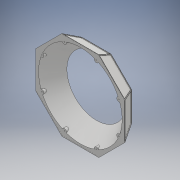
# Autodesk Inventor part: meteostanica radiation shield zakladna
Saved by Autodesk Inventor 2017 (Build 210142000, 142)
## iProperties
Created: 2017-02-23
Part Number: meteostanica radiation shield zakladna
Material: Generic
Document SubType Name: Modeling
Designer: Luc3as
Density: 1 g/cm^3
Appearance: Default
Author: Luc3as
Autodesk Inventor part; units mm, degrees
ref_plane "YZ Plane" through (0, 0, 0) normal (1, 0, 0) x (0, 1, 0)
ref_plane "XZ Plane" through (0, 0, 0) normal (0, 1, 0) x (-1, 0, 0)
ref_plane "XY Plane" through (0, 0, 0) normal (0, 0, 1) x (1, 0, 0)
sketch "Sketch1" plane through (0, 0, 0) normal (0, 1, 0) x (-1, 0, 0)
  circle A0 centre (0, 0) radius 75
  line L0 (82.6875, -34.2503) -> (34.2503, -82.6875)
  line L1 (34.2503, -82.6875) -> (-34.2503, -82.6875)
  line L2 (-34.2503, -82.6875) -> (-82.6875, -34.2503)
  line L3 (-82.6875, -34.2503) -> (-82.6875, 34.2503)
  line L4 (-82.6875, 34.2503) -> (-34.2503, 82.6875)
  line L5 (-34.2503, 82.6875) -> (34.2503, 82.6875)
  line L6 (34.2503, 82.6875) -> (82.6875, 34.2503)
  line L7 (82.6875, 34.2503) -> (82.6875, -34.2503)
  circle A1 centre (0, 0) radius 55
  line L8 (63.0062, -26.098) -> (26.098, -63.0062)
  line L9 (26.098, -63.0062) -> (-26.098, -63.0062)
  line L10 (-26.098, -63.0062) -> (-63.0062, -26.098)
  line L11 (-63.0062, -26.098) -> (-63.0062, 26.098)
  line L12 (-63.0062, 26.098) -> (-26.098, 63.0062)
  line L13 (-26.098, 63.0062) -> (26.098, 63.0062)
  line L14 (26.098, 63.0062) -> (63.0062, 26.098)
  line L15 (63.0062, 26.098) -> (63.0062, -26.098)
  point P0 (75, 0)
  dimension "d0" = 150
  dimension "d1" = 110
  constraints: 32 end point, 3 coincident, 1 centre point, 1 horizontal alignment, 3 other
  measures "d1" diameter of A1
extrude "Extrusion1" add sketch "Sketch1" along normal blind 30 contours A0 | L0 L1 L2 L3 L4 L5 L6 L7 | L8 L9 L10 L11 L12 L13 L14 L15
draft "FaceDraft1" angle 30 pull direction (0, 1, 0) faces at (-50.396, 20, 66.5418) (11.4168, 20, 82.6875) (66.5418, 20, 50.396) (-82.6875, 10, 11.4168) (-66.5418, 10, -50.396) (-11.4168, 10, -82.6875) (50.396, 10, -66.5418) (82.6875, 10, -11.4168) fixed edges at (-58.4689, 0, 58.4689) (0, 0, 82.6875) (58.4689, 0, 58.4689) (-82.6875, 0, 0) (-58.4689, 0, -58.4689) (0, 0, -82.6875) (58.4689, 0, -58.4689) (82.6875, 0, 0)
sketch "Sketch2" plane through (82.6875, 0, -34.2503) normal (0.6123724, 0.5, -0.6123724) x (-0.7071068, 0, -0.7071068)
  line L0 (68.5006, 0) -> (0, 0) projected
  line L1 (34.2503, 0) -> (61.2503, 0)
  line L2 (61.2503, 0) -> (61.2503, 27)
  line L3 (61.2503, 27) -> (7.2503, 27)
  line L4 (7.2503, 27) -> (7.2503, 0)
  line L5 (7.2503, 0) -> (34.2503, 0)
  line L6 (68.5006, 0) -> (61.3262, 34.641) projected
  line L7 (68.5006, 0) -> (0, 0) projected
  line L8 (68.5006, 0) -> (61.3262, 34.641) projected
  line L9 (7.1744, 34.641) -> (61.3262, 34.641) projected
  line L10 (0, 0) -> (7.1744, 34.641) projected
  line L11 (60.5121, 33.641) -> (67.2722, 1)
  line L12 (67.2722, 1) -> (1.2283, 1)
  line L13 (1.2283, 1) -> (7.9885, 33.641)
  line L14 (7.9885, 33.641) -> (60.5121, 33.641)
  point P0 (34.2503, 41.3438)
  dimension "d5" = 27
  dimension "d6" = 27
  dimension "d7" = 54
  dimension "d10" = 1
  constraints: 18 end point, 4 perpendicular, 2 point on line, 1 midpoint, 3 other
  measures "d5" distance of L1.start L1.end
  measures "d6" distance of L1.end L2.end
  measures "d7" distance of L2.end L3.end
  measures "d10" distance between parallel lines of L9 L14
draft "FaceDraft2" angle 37 pull direction (0, -1, 0) faces at (50.386, 20, -22.0512) fixed edges at (55, 30, 0)
sketch "Sketch3" plane through (82.6875, 0, 34.2503) normal (0.8660254, 0.5, 0) x (0, 0, -1)
  line L0 (7.1744, 34.641) -> (61.3262, 34.641) projected
  line L1 (68.5006, 0) -> (0, 0) projected
  line L2 (68.5006, 0) -> (61.3262, 34.641) projected
  line L3 (7.1744, 34.641) -> (61.3262, 34.641) projected
  line L4 (0, 0) -> (7.1744, 34.641) projected
  line L5 (60.5121, 33.641) -> (67.2722, 1)
  line L6 (67.2722, 1) -> (1.2283, 1)
  line L7 (1.2283, 1) -> (7.9885, 33.641)
  line L8 (7.9885, 33.641) -> (60.5121, 33.641)
  point P0 (34.2503, 41.3437)
  dimension "d9" = 1
  constraints: 8 end point, 3 other
  measures "d9" distance between parallel lines of L2 L5
sketch "Sketch4" plane through (82.6875, 0, -34.2503) normal (0.6123724, 0.5, -0.6123724) x (-0.7071068, 0, -0.7071068)
  point P0 (34.2503, 41.3438)
sketch "Sketch5" plane through (34.2503, 0, -82.6875) normal (0, 0.5, -0.8660254) x (-1, 0, 0)
  line L0 (7.1744, 34.641) -> (61.3262, 34.641) projected
  line L1 (68.5006, 0) -> (0, 0) projected
  line L2 (68.5006, 0) -> (61.3262, 34.641) projected
  line L3 (7.1744, 34.641) -> (61.3262, 34.641) projected
  line L4 (0, 0) -> (7.1744, 34.641) projected
  line L5 (7.9885, 33.641) -> (60.5121, 33.641)
  line L6 (60.5121, 33.641) -> (67.2722, 1)
  line L7 (67.2722, 1) -> (1.2283, 1)
  line L8 (1.2283, 1) -> (7.9885, 33.641)
  point P0 (34.2503, 41.3438)
  dimension "d11" = 1
  constraints: 8 end point, 3 other
  measures "d11" distance between parallel lines of L4 L8
sketch "Sketch6" plane through (34.2503, 0, 82.6875) normal (0.6123724, 0.5, 0.6123724) x (0.7071068, 0, -0.7071068)
  line L0 (7.1744, 34.641) -> (61.3262, 34.641) projected
  line L1 (68.5006, 0) -> (0, 0) projected
  line L2 (68.5006, 0) -> (61.3262, 34.641) projected
  line L3 (7.1744, 34.641) -> (61.3262, 34.641) projected
  line L4 (0, 0) -> (7.1744, 34.641) projected
  line L5 (7.9885, 33.641) -> (60.5121, 33.641)
  line L6 (60.5121, 33.641) -> (67.2722, 1)
  line L7 (67.2722, 1) -> (1.2283, 1)
  line L8 (1.2283, 1) -> (7.9885, 33.641)
  point P0 (34.2503, 41.3437)
  dimension "d12" = 1
  constraints: 8 end point, 3 other
  measures "d12" distance between parallel lines of L4 L8
sketch "Sketch7" plane through (-34.2503, 0, -82.6875) normal (-0.6123724, 0.5, -0.6123724) x (-0.7071068, 0, 0.7071068)
  line L0 (68.5006, 0) -> (61.3262, 34.641) projected
  line L1 (68.5006, 0) -> (0, 0) projected
  line L2 (68.5006, 0) -> (61.3262, 34.641) projected
  line L3 (7.1744, 34.641) -> (61.3262, 34.641) projected
  line L4 (0, 0) -> (7.1744, 34.641) projected
  line L5 (60.5121, 33.641) -> (67.2722, 1)
  line L6 (67.2722, 1) -> (1.2283, 1)
  line L7 (1.2283, 1) -> (7.9885, 33.641)
  line L8 (7.9885, 33.641) -> (60.5121, 33.641)
  point P0 (34.2503, 41.3438)
  dimension "d13" = 1
  constraints: 8 end point, 3 other
  measures "d13" distance between parallel lines of L3 L8
sketch "Sketch8" plane through (-82.6875, 0, -34.2503) normal (-0.8660254, 0.5, 0) x (0, 0, 1)
  line L0 (68.5006, 0) -> (61.3262, 34.641) projected
  line L1 (68.5006, 0) -> (0, 0) projected
  line L2 (68.5006, 0) -> (61.3262, 34.641) projected
  line L3 (7.1744, 34.641) -> (61.3262, 34.641) projected
  line L4 (0, 0) -> (7.1744, 34.641) projected
  line L5 (60.5121, 33.641) -> (67.2722, 1)
  line L6 (67.2722, 1) -> (1.2283, 1)
  line L7 (1.2283, 1) -> (7.9885, 33.641)
  line L8 (7.9885, 33.641) -> (60.5121, 33.641)
  point P0 (34.2503, 41.3438)
  dimension "d14" = 1
  constraints: 8 end point, 3 other
  measures "d14" distance between parallel lines of L3 L8
sketch "Sketch9" plane through (-82.6875, 0, 34.2503) normal (-0.6123724, 0.5, 0.6123724) x (0.7071068, 0, 0.7071068)
  line L0 (68.5006, 0) -> (61.3262, 34.641) projected
  line L1 (68.5006, 0) -> (0, 0) projected
  line L2 (68.5006, 0) -> (61.3262, 34.641) projected
  line L3 (7.1744, 34.641) -> (61.3262, 34.641) projected
  line L4 (0, 0) -> (7.1744, 34.641) projected
  line L5 (1.2283, 1) -> (67.2722, 1)
  line L6 (67.2722, 1) -> (60.5121, 33.641)
  line L7 (60.5121, 33.641) -> (7.9885, 33.641)
  line L8 (7.9885, 33.641) -> (1.2283, 1)
  point P0 (34.2503, 41.3437)
  dimension "d15" = 1
  constraints: 8 end point, 3 other
  measures "d15" distance between parallel lines of L1 L5
sketch "Sketch10" plane through (-34.2503, 0, 82.6875) normal (0, 0.5, 0.8660254) x (1, 0, 0)
  line L0 (68.5006, 0) -> (0, 0) projected
  line L1 (68.5006, 0) -> (0, 0) projected
  line L2 (68.5006, 0) -> (61.3262, 34.641) projected
  line L3 (7.1744, 34.641) -> (61.3262, 34.641) projected
  line L4 (0, 0) -> (7.1744, 34.641) projected
  line L5 (60.5121, 33.641) -> (67.2722, 1)
  line L6 (67.2722, 1) -> (1.2283, 1)
  line L7 (1.2283, 1) -> (7.9885, 33.641)
  line L8 (7.9885, 33.641) -> (60.5121, 33.641)
  point P0 (34.2503, 41.3437)
  dimension "d16" = 1
  constraints: 8 end point, 3 other
  measures "d16" distance between parallel lines of L2 L5
extrude "Extrusion2" cut sketch "Sketch5" against normal blind 1 contours L5 L6 L7 L8
extrude "Extrusion3" cut sketch "Sketch7" against normal blind 1 contours L5 L6 L7 L8
extrude "Extrusion4" cut sketch "Sketch8" against normal blind 1 contours L5 L6 L7 L8
extrude "Extrusion5" cut sketch "Sketch9" against normal blind 1 contours L8 L7 L6 L5
extrude "Extrusion6" cut sketch "Sketch10" against normal blind 1 contours L5 L6 L7 L8
extrude "Extrusion7" cut sketch "Sketch6" against normal blind 1 contours L5 L6 L7 L8
extrude "Extrusion8" cut sketch "Sketch3" against normal blind 1 contours L5 L6 L7 L8
extrude "Extrusion9" cut sketch "Sketch2" against normal blind 1 contours L12 L4 L3 L2 | L2 L3 L4 L12 L13 L14 L11
sketch "Sketch11" plane through (0, 0, 0) normal (0, -1, 0) x (1, 0, 0)
  line L0 (-34.2503, 82.6875) -> (-82.6875, 34.2503) projected
  line L1 (-82.6875, -34.2503) -> (-34.2503, -82.6875) projected
  line L2 (-34.2503, -82.6875) -> (34.2503, -82.6875) projected
  line L3 (34.2503, -82.6875) -> (82.6875, -34.2503) projected
  line L4 (82.6875, -34.2503) -> (82.6875, 34.2503) projected
  line L5 (82.6875, 34.2503) -> (34.2503, 82.6875) projected
  line L6 (34.2503, 82.6875) -> (-34.2503, 82.6875) projected
  line L7 (-34.2503, 82.6875) -> (-82.6875, 34.2503) projected
  line L8 (-82.6875, 34.2503) -> (-82.6875, -34.2503) projected
  line L9 (82.6875, 34.2503) -> (34.2503, 82.6875) projected
  line L10 (-80.853, 34.1529) -> (-64.5325, 27.3927) projected
  line L11 (81.3215, 33.022) -> (65.001, 26.2618) projected
  circle A0 centre (71.6992, 29.6988) radius 4
  circle A1 centre (71.6992, -29.6988) radius 4
  circle A2 centre (29.6988, -71.6992) radius 4
  circle A3 centre (-29.6988, -71.6992) radius 4
  circle A4 centre (-71.6992, -29.6988) radius 4
  circle A5 centre (-71.6992, 29.6988) radius 4
  circle A6 centre (-29.6988, 71.6992) radius 4
  circle A7 centre (29.6988, 71.6992) radius 4
  dimension "d35" = 8
  dimension "d36" = 8
  dimension "d37" = 8
  dimension "d38" = 8
  dimension "d39" = 8
  dimension "d40" = 8
  dimension "d41" = 8
  dimension "d42" = 8
  constraints: 8 centre point
  measures "d35" diameter of A0
  measures "d36" diameter of A1
  measures "d37" diameter of A2
  measures "d38" diameter of A3
  measures "d39" diameter of A4
  measures "d40" diameter of A5
  measures "d41" diameter of A6
  measures "d42" diameter of A7
extrude "Extrusion10" add sketch "Sketch11" against normal up to next contours A5 L10 | L10 A5 | A0 L11 | L11 A0 | A1 | A2 | A3 | A4 | A6 | A7
sketch "Sketch12" plane through (0, 0, 0) normal (0, -1, 0) x (1, 0, 0)
  arc A0 (25.965, 73.1342) -> (33.3536, 70.0737) centre (29.6988, 71.6992) ccw projected
  arc A1 (-33.3536, 70.0737) -> (-25.965, 73.1342) centre (-29.6988, 71.6992) ccw projected
  arc A2 (70.0737, 33.3536) -> (73.1342, 25.965) centre (71.6992, 29.6988) ccw projected
  arc A3 (73.1342, -25.965) -> (70.0737, -33.3536) centre (71.6992, -29.6988) ccw projected
  line L0 (-82.6875, -34.2503) -> (-34.2503, -82.6875) projected
  line L1 (-34.2503, -82.6875) -> (34.2503, -82.6875) projected
  line L2 (34.2503, -82.6875) -> (82.6875, -34.2503) projected
  line L3 (82.6875, -34.2503) -> (82.6875, 34.2503) projected
  line L4 (82.6875, 34.2503) -> (34.2503, 82.6875) projected
  line L5 (34.2503, 82.6875) -> (-34.2503, 82.6875) projected
  line L6 (-34.2503, 82.6875) -> (-82.6875, 34.2503) projected
  line L7 (-82.6875, 34.2503) -> (-82.6875, -34.2503) projected
  arc A4 (-33.3536, 70.0737) -> (-25.965, 73.1342) centre (-29.6988, 71.6992) ccw projected
  arc A5 (25.965, 73.1342) -> (-25.965, 73.1342) centre (0, 0) ccw projected
  arc A6 (25.965, 73.1342) -> (33.3536, 70.0737) centre (29.6988, 71.6992) ccw projected
  arc A7 (70.0737, 33.3536) -> (33.3536, 70.0737) centre (0, 0) ccw projected
  arc A8 (70.0737, 33.3536) -> (73.1342, 25.965) centre (71.6992, 29.6988) ccw projected
  arc A9 (73.1342, -25.965) -> (73.1342, 25.965) centre (0, 0) ccw projected
  arc A10 (73.1342, -25.965) -> (70.0737, -33.3536) centre (71.6992, -29.6988) ccw projected
  arc A11 (33.3536, -70.0737) -> (70.0737, -33.3536) centre (0, 0) ccw projected
  arc A12 (33.3536, -70.0737) -> (25.965, -73.1342) centre (29.6988, -71.6992) ccw projected
  arc A13 (-25.965, -73.1342) -> (25.965, -73.1342) centre (0, 0) ccw projected
  arc A14 (-25.965, -73.1342) -> (-33.3536, -70.0737) centre (-29.6988, -71.6992) ccw projected
  arc A15 (-70.0737, -33.3536) -> (-33.3536, -70.0737) centre (0, 0) ccw projected
  arc A16 (-70.0737, -33.3536) -> (-73.1342, -25.965) centre (-71.6992, -29.6988) ccw projected
  arc A17 (-73.1342, 25.965) -> (-73.1342, -25.965) centre (0, 0) ccw projected
  arc A18 (-73.1342, 25.965) -> (-70.0737, 33.3536) centre (-71.6992, 29.6988) ccw projected
  arc A19 (-33.3536, 70.0737) -> (-70.0737, 33.3536) centre (0, 0) ccw projected
hole "Hole1" at (29.6988, 0, 71.6992) at (-29.6988, 0, 71.6992) at (71.6992, 0, 29.6988) at (71.6992, 0, -29.6988) at (29.6988, 0, -71.6992) at (-29.6988, 0, -71.6992) at (-71.6992, 0, -29.6988) at (-71.6992, 0, 29.6988) direction (0, 1, 0) diameter 1.5 depth 13 tip angle 118
body "Solid1"
